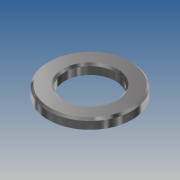
# Autodesk Inventor part: DD_KVD_003_10_C
Saved by Autodesk Inventor 2017.3 (Build 213256000, 256)
## iProperties
Created: 2023-12-12
Part Number: DD_KVD_003_10_C
Material: Nerezová ocel
Document SubType Name: Modeling
Designer: Darena
Manufacturer: Standard
Standards Organization: Custom
Density: 8 g/cm^3
Appearance: Pololeštěná
Author: Darena
Autodesk Inventor part; units mm, degrees
ref_plane "YZ Plane" through (0, 0, 0) normal (1, 0, 0) x (0, 1, 0)
ref_plane "XZ Plane" through (0, 0, 0) normal (0, 1, 0) x (-1, 0, 0)
ref_plane "XY Plane" through (0, 0, 0) normal (0, 0, 1) x (1, 0, 0)
sketch "Náčrt2" plane through (0, 0, 0) normal (1, 0, 0) x (0, 1, 0)
  line L0 (0, 0) -> (11, 0)
  line L1 (11, 0) -> (11, -2.5)
  line L2 (11, -2.5) -> (0, -2.5)
  line L3 (0, 0) -> (0, -2.5)
  line L4 (6.6, 0) -> (6.6, -2.5)
  dimension "d3" = 2.5
  dimension "d13" = 22
  dimension "d14" = 13.2
  constraints: 10 end point, 3 perpendicular, 2 horizontal, 2 point on line, 1 vertical
  measures "d3" distance between parallel lines of L2 L0
  measures "d13" diameter of L1 L3
  measures "d14" diameter of L4 L3
revolve "Rotace1" add sketch "Náčrt2" angle 360 about axis through (0, 0, 0) along (0, 0, -1) contours L0 L1 L2 L4
chamfer "Zkosení1" distance 0.5 angle 45 2 edges at (0, -11, 0) (0, -6.6, 0)
